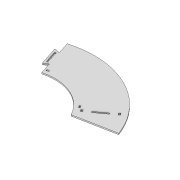
# Autodesk Inventor part: Level 1d - V2
Saved by Autodesk Inventor 2020 (Build 240168000, 168)
## iProperties
Created: 2020-07-30
Part Number: Level 1d - V2
Material: Generic
Document SubType Name: Modeling
Designer: Dan Wikman
Density: 1 g/cm^3
Appearance: Default
Author: Dan Wikman
Autodesk Inventor part; units mm, degrees
ref_plane "YZ Plane" through (0, 0, 0) normal (1, 0, 0) x (0, 1, 0)
ref_plane "XZ Plane" through (0, 0, 0) normal (0, 1, 0) x (-1, 0, 0)
ref_plane "XY Plane" through (0, 0, 0) normal (0, 0, 1) x (1, 0, 0)
sketch "Sketch1" plane through (0, 0, 0) normal (0, 1, 0) x (-1, 0, 0)
  line L0 (0, 0) -> (618.944217, 0)
  line L1 (0, 0) -> (191.264282, 588.650931)
  line L2 (0, 0) -> (-500.73639, 363.806283)
  line L3 (0, 0) -> (-500.73639, -363.806283)
  line L4 (0, 0) -> (191.264282, -588.650931)
  line L5 (396.643783, 3.75) -> (328.143784, 3.75)
  line L6 (328.143784, -3.75) -> (396.643784, -3.75)
  arc A0 (472.393783, 0) -> (145.977707, 449.273186) centre (0, 0) ccw
  arc A1 (77.993968, -240.040752) -> (252.393783, 0) centre (0, 0) ccw
  line L7 (289.893785, 3.75) -> (283.893784, 3.75)
  line L8 (283.893783, -3.75) -> (289.893781, -3.75)
  arc A2 (328.143784, 3.75) -> (326.393783, 2) centre (328.143783, 2) ccw
  arc A3 (326.393783, -1.999999) -> (328.143784, -3.75) centre (328.143783, -2) ccw
  line L9 (326.393783, 2) -> (326.393783, -1.999999)
  arc A4 (398.393783, 2) -> (396.643783, 3.75) centre (396.643783, 2) ccw
  arc A5 (396.643784, -3.75) -> (398.393783, -2.013555) centre (396.657285, -2.013555) ccw
  line L10 (398.393783, -2.013555) -> (398.393783, 2)
  line L11 (362.393784, -3.75) -> (362.393784, 32.980572)
  arc A6 (283.893784, 3.75) -> (282.143784, 2) centre (283.893784, 2) ccw
  arc A7 (282.143784, -2) -> (283.893783, -3.75) centre (283.893784, -2) ccw
  arc A8 (289.893781, -3.75) -> (291.643782, -2.000001) centre (289.893781, -2) ccw
  arc A9 (291.643784, 1.999999) -> (289.893785, 3.75) centre (289.893785, 2) ccw
  line L12 (291.643784, 1.999999) -> (291.643782, -2.000001)
  line L13 (282.143784, -2) -> (282.143784, 2)
  line L14 (434.893784, 3.75) -> (440.893785, 3.75)
  line L15 (440.893786, -3.75) -> (434.893788, -3.75)
  arc A10 (442.643785, 2) -> (440.893785, 3.75) centre (440.893785, 2) ccw
  arc A11 (440.893786, -3.75) -> (442.643785, -2) centre (440.893785, -2) ccw
  arc A12 (433.143787, -2.000001) -> (434.893788, -3.75) centre (434.893788, -2) ccw
  arc A13 (434.893784, 3.75) -> (433.143785, 1.999999) centre (434.893784, 2) ccw
  line L16 (433.143785, 1.999999) -> (433.143787, -2.000001)
  line L17 (442.643785, -2) -> (442.643785, 2)
  line L18 (131.946679, 412.562253) -> (135.750905, 411.326187)
  arc A14 (130.823108, 414.767381) -> (131.946679, 412.562253) centre (132.487457, 414.226602) ccw
  arc A15 (135.750905, 411.326187) -> (137.956033, 412.449757) centre (136.291684, 412.990537) ccw
  line L19 (139.810135, 418.156094) -> (137.956033, 412.449757)
  line L20 (130.823108, 414.767381) -> (132.67721, 420.473721)
  arc A16 (134.882339, 421.59729) -> (132.67721, 420.473721) centre (134.341559, 419.932941) ccw
  line L21 (138.686565, 420.361222) -> (134.882339, 421.59729)
  arc A17 (139.810135, 418.156094) -> (138.686565, 420.361222) centre (138.145785, 418.696873) ccw
  line L22 (125.025454, 378.272781) -> (121.208336, 379.513038)
  arc A18 (121.208336, 379.513038) -> (119.003208, 378.389469) centre (120.667557, 377.848689) ccw
  arc A19 (126.136132, 376.071842) -> (125.025454, 378.272781) centre (124.488846, 376.621273) ccw
  line L23 (119.003208, 378.389469) -> (97.835544, 313.242097)
  line L24 (98.959113, 311.036969) -> (102.763338, 309.800901)
  arc A20 (97.835544, 313.242097) -> (98.959113, 311.036969) centre (99.499893, 312.701317) ccw
  arc A21 (102.763338, 309.800901) -> (104.968468, 310.924471) centre (103.304119, 311.465249) ccw
  line L25 (104.968468, 310.924471) -> (126.136132, 376.071842)
  line L26 (88.220774, 277.987755) -> (92.024998, 276.751685)
  arc A22 (93.148567, 274.546556) -> (92.024998, 276.751685) centre (91.484218, 275.087336) ccw
  line L27 (91.294465, 268.840219) -> (93.148567, 274.546556)
  arc A23 (88.220774, 277.987755) -> (86.015644, 276.864187) centre (87.679993, 276.323407) ccw
  line L28 (86.015644, 276.864187) -> (84.161542, 271.157847)
  arc A24 (84.161542, 271.157847) -> (85.285111, 268.952718) centre (85.825891, 270.617067) ccw
  arc A25 (89.089337, 267.71665) -> (91.294465, 268.840219) centre (89.630117, 269.380999) ccw
  line L29 (89.089337, 267.71665) -> (85.285111, 268.952718)
  line L30 (-351.596253, 252.977496) -> (-349.245114, 256.213565)
  arc A26 (-354.040657, 252.590339) -> (-351.596253, 252.977496) centre (-353.012033, 254.006119) ccw
  arc A27 (-349.245114, 256.213565) -> (-349.63227, 258.657968) centre (-350.660895, 257.242188) ccw
  line L31 (-354.486371, 262.184679) -> (-349.63227, 258.657968)
  line L32 (-354.040657, 252.590339) -> (-358.89476, 256.117051)
  arc A28 (-359.281915, 258.561455) -> (-358.89476, 256.117051) centre (-357.866135, 257.532831) ccw
  line L33 (-356.930774, 261.797523) -> (-359.281915, 258.561455)
  arc A29 (-354.486371, 262.184679) -> (-356.930774, 261.797523) centre (-355.514994, 260.768899) ccw
  line L34 (-321.123804, 235.79899) -> (-323.482912, 232.551956)
  arc A30 (-323.482912, 232.551956) -> (-323.095756, 230.107553) centre (-322.067132, 231.523332) ccw
  arc A31 (-318.687368, 236.175181) -> (-321.123804, 235.79899) centre (-319.718947, 234.778302) ccw
  line L35 (-323.095756, 230.107553) -> (-267.678092, 189.844263)
  line L36 (-265.233688, 190.231418) -> (-262.882548, 193.467485)
  arc A32 (-267.678092, 189.844263) -> (-265.233688, 190.231418) centre (-266.649468, 191.260043) ccw
  arc A33 (-262.882548, 193.467485) -> (-263.269704, 195.911891) centre (-264.298327, 194.496111) ccw
  line L37 (-263.269704, 195.911891) -> (-318.687368, 236.175181)
  line L38 (-237.120347, 169.805882) -> (-234.769205, 173.041948)
  arc A34 (-232.324801, 173.429103) -> (-234.769205, 173.041948) centre (-233.353425, 172.013323) ccw
  line L39 (-227.4707, 169.902393) -> (-232.324801, 173.429103)
  arc A35 (-237.120347, 169.805882) -> (-236.733193, 167.361478) centre (-235.704569, 168.777257) ccw
  line L40 (-236.733193, 167.361478) -> (-231.87909, 163.834766)
  arc A36 (-231.87909, 163.834766) -> (-229.434686, 164.221921) centre (-230.850466, 165.250545) ccw
  arc A37 (-227.083545, 167.457989) -> (-227.4707, 169.902393) centre (-228.499325, 168.486613) ccw
  line L41 (-227.083545, 167.457989) -> (-229.434686, 164.221921)
  line L42 (-349.245113, -256.213562) -> (-351.596256, -252.977496)
  arc A38 (-349.632267, -258.657966) -> (-349.245113, -256.213562) centre (-350.660892, -257.242187) ccw
  arc A39 (-351.596256, -252.977496) -> (-354.04066, -252.590341) centre (-353.012035, -254.006121) ccw
  line L43 (-358.89476, -256.117051) -> (-354.04066, -252.590341)
  line L44 (-349.632267, -258.657966) -> (-354.48637, -262.184678)
  arc A40 (-356.930774, -261.797523) -> (-354.48637, -262.184678) centre (-355.514994, -260.768899) ccw
  line L45 (-359.281915, -258.561455) -> (-356.930774, -261.797523)
  arc A41 (-358.89476, -256.117051) -> (-359.281915, -258.561455) centre (-357.866135, -257.532831) ccw
  line L46 (-323.490879, -232.540991) -> (-321.131771, -235.788024)
  arc A42 (-321.131771, -235.788024) -> (-318.687367, -236.17518) centre (-319.715991, -234.7594) ccw
  arc A43 (-323.095757, -230.107553) -> (-323.490879, -232.540991) centre (-322.086023, -231.520303) ccw
  line L47 (-318.687367, -236.17518) -> (-263.269703, -195.91189)
  line L48 (-262.882547, -193.467486) -> (-265.233687, -190.231419)
  arc A44 (-263.269703, -195.91189) -> (-262.882547, -193.467486) centre (-264.298327, -194.496111) ccw
  arc A45 (-265.233687, -190.231419) -> (-267.678093, -189.844263) centre (-266.649468, -191.260043) ccw
  line L49 (-267.678093, -189.844263) -> (-323.095757, -230.107553)
  line L50 (-234.769208, -173.041948) -> (-237.120347, -169.805879)
  arc A46 (-236.73319, -167.361476) -> (-237.120347, -169.805879) centre (-235.704566, -168.777256) ccw
  line L51 (-231.87909, -163.834765) -> (-236.73319, -167.361476)
  arc A47 (-234.769208, -173.041948) -> (-232.324804, -173.429105) centre (-233.353428, -172.013326) ccw
  line L52 (-232.324804, -173.429105) -> (-227.470701, -169.902393)
  arc A48 (-227.470701, -169.902393) -> (-227.083545, -167.457989) centre (-228.499325, -168.486613) ccw
  arc A49 (-229.434686, -164.221921) -> (-231.87909, -163.834765) centre (-230.850466, -165.250545) ccw
  line L53 (-229.434686, -164.221921) -> (-227.083545, -167.457989)
  line L54 (135.750902, -411.326185) -> (131.946678, -412.562255)
  arc A50 (137.956032, -412.449754) -> (135.750902, -411.326185) centre (136.291683, -412.990533) ccw
  arc A51 (131.946678, -412.562255) -> (130.823109, -414.767384) centre (132.487459, -414.226604) ccw
  line L55 (132.677211, -420.473722) -> (130.823109, -414.767384)
  line L56 (137.956032, -412.449754) -> (139.810134, -418.156094)
  arc A52 (138.686565, -420.361222) -> (139.810134, -418.156094) centre (138.145785, -418.696873) ccw
  line L57 (134.882339, -421.59729) -> (138.686565, -420.361222)
  arc A53 (132.677211, -420.473722) -> (134.882339, -421.59729) centre (134.341559, -419.932941) ccw
  line L58 (121.195445, -379.517226) -> (125.012563, -378.27697)
  arc A54 (125.012563, -378.27697) -> (126.136132, -376.071841) centre (124.471783, -376.612621) ccw
  arc A55 (119.003208, -378.38947) -> (121.195445, -379.517226) centre (120.658838, -377.865719) ccw
  line L59 (126.136132, -376.071841) -> (104.968468, -310.92447)
  line L60 (102.763339, -309.800901) -> (98.959114, -311.036968)
  arc A56 (104.968468, -310.92447) -> (102.763339, -309.800901) centre (103.304119, -311.465249) ccw
  arc A57 (98.959114, -311.036968) -> (97.835544, -313.242098) centre (99.499893, -312.701317) ccw
  line L61 (97.835544, -313.242098) -> (119.003208, -378.38947)
  line L62 (92.024997, -276.751688) -> (88.220771, -277.987753)
  arc A58 (86.015643, -276.864184) -> (88.220771, -277.987753) centre (87.679992, -276.323404) ccw
  line L63 (84.161542, -271.157846) -> (86.015643, -276.864184)
  arc A59 (92.024997, -276.751688) -> (93.148568, -274.546559) centre (91.484219, -275.087339) ccw
  line L64 (93.148568, -274.546559) -> (91.294466, -268.840219)
  arc A60 (91.294466, -268.840219) -> (89.089337, -267.71665) centre (89.630117, -269.380999) ccw
  arc A61 (85.285111, -268.952718) -> (84.161542, -271.157846) centre (85.825891, -270.617067) ccw
  line L65 (85.285111, -268.952718) -> (89.089337, -267.71665)
  line L66 (-442.530326, 165.296089) -> (-220.837003, 122.203273)
  line L67 (-442.530326, -165.296089) -> (-220.837003, -122.203273)
  arc A62 (252.393783, 0) -> (-220.837003, 122.203273) centre (0, 0) ccw
  arc A63 (-220.837003, -122.203273) -> (77.993968, -240.040752) centre (0, 0) ccw
  arc A64 (145.977707, 449.273186) -> (-442.530326, 165.296089) centre (0, 0) ccw
  arc A65 (-442.530326, -165.296089) -> (472.393783, 0) centre (0, 0) ccw
  line L68 (115.678154, 400.516685) -> (82.986198, 299.90119)
  line L69 (84.650547, 297.61041) -> (108.748421, 297.61041)
  line L70 (110.41277, 295.31963) -> (90.955171, 235.435297)
  line L71 (138.866228, 382.890368) -> (158.992883, 444.833845)
  line L72 (118.634381, 401.156393) -> (135.910001, 382.25066)
  line L73 (123.116895, 378.892909) -> (127.272191, 391.703526) construction
  line L74 (100.861225, 310.418935) -> (96.699484, 297.61041) construction
  arc A66 (135.910001, 382.25066) -> (138.866228, 382.890368) centre (137.201879, 383.431148) ccw
  arc A67 (118.634381, 401.156393) -> (115.678154, 400.516685) centre (117.342503, 399.975905) ccw
  arc A68 (82.986198, 299.90119) -> (84.650547, 297.61041) centre (84.650547, 299.36041) ccw
  arc A69 (110.41277, 295.31963) -> (108.748421, 297.61041) centre (108.748421, 295.86041) ccw
  line L75 (407.062404, -13.75) -> (472.19363, -13.75)
  arc A70 (405.540481, -11.136142) -> (407.062404, -13.75) centre (407.062404, -12) ccw
  line L76 (418.182442, 11.136142) -> (405.540481, -11.136142)
  arc A71 (418.182442, 11.136142) -> (416.660519, 13.75) centre (416.660519, 12) ccw
  line L77 (416.660519, 13.75) -> (310.867126, 13.75)
  line L78 (309.202778, 11.45922) -> (316.64943, -11.45922)
  arc A72 (310.867126, 13.75) -> (309.202778, 11.45922) centre (310.867126, 12) ccw
  arc A73 (314.985081, -13.75) -> (316.64943, -11.45922) centre (314.985081, -12) ccw
  line L79 (314.985081, -13.75) -> (252.018966, -13.75)
  line L80 (112.712173, -391.388335) -> (132.838829, -453.331812)
  arc A74 (114.7278, -389.133174) -> (112.712173, -391.388335) centre (114.376522, -390.847556) ccw
  line L81 (139.816582, -394.273879) -> (114.7278, -389.133174)
  arc A75 (139.816582, -394.273879) -> (141.832208, -392.018718) centre (140.167859, -392.559497) ccw
  line L82 (141.832208, -392.018718) -> (109.140252, -291.403223)
  line L83 (106.447279, -290.528223) -> (86.951689, -304.692598)
  arc A76 (109.140252, -291.403223) -> (106.447279, -290.528223) centre (107.475903, -291.944002) ccw
  arc A77 (84.258716, -303.817598) -> (86.951689, -304.692598) centre (85.923065, -303.276818) ccw
  line L84 (84.258716, -303.817598) -> (64.801116, -243.933264)
  line L85 (277, 35.5) -> (273, 35.5)
  line L86 (271.25, 33.75) -> (271.25, 23.75)
  line L87 (273, 22) -> (277, 22)
  line L88 (278.75, 23.75) -> (278.75, 33.75)
  arc A78 (278.75, 33.75) -> (277, 35.5) centre (277, 33.75) ccw
  arc A79 (273, 35.5) -> (271.25, 33.75) centre (273, 33.75) ccw
  arc A80 (271.25, 23.75) -> (273, 22) centre (273, 23.75) ccw
  arc A81 (277, 22) -> (278.75, 23.75) centre (277, 23.75) ccw
  line L89 (277, -35.5) -> (273, -35.5)
  line L90 (271.25, -33.75) -> (271.25, -23.75)
  line L91 (273, -22) -> (277, -22)
  line L92 (278.75, -23.75) -> (278.75, -33.75)
  arc A82 (277, -35.5) -> (278.75, -33.75) centre (277, -33.75) ccw
  arc A83 (271.25, -33.75) -> (273, -35.5) centre (273, -33.75) ccw
  arc A84 (273, -22) -> (271.25, -23.75) centre (273, -23.75) ccw
  arc A85 (278.75, -23.75) -> (277, -22) centre (277, -23.75) ccw
  arc A86 (64.674464, 270.241029) -> (63.550895, 272.446158) centre (63.010115, 270.781809) ccw
  line L93 (63.550895, 272.446158) -> (54.04033, 275.536327)
  line L94 (63.438396, 266.436803) -> (64.674464, 270.241029)
  arc A87 (61.233267, 265.313234) -> (63.438396, 266.436803) centre (61.774047, 266.977583) ccw
  line L95 (51.835201, 274.412758) -> (50.599133, 270.608532)
  line L96 (51.722702, 268.403404) -> (61.233267, 265.313234)
  arc A88 (50.599133, 270.608532) -> (51.722702, 268.403404) centre (52.263482, 270.067753) ccw
  arc A89 (54.04033, 275.536327) -> (51.835201, 274.412758) centre (53.49955, 273.871979) ccw
  arc A90 (108.726079, 257.76785) -> (106.520951, 256.644281) centre (108.1853, 256.103501) ccw
  line L97 (105.284883, 252.840055) -> (106.520951, 256.644281)
  arc A91 (105.284883, 252.840055) -> (106.408452, 250.634926) centre (106.949232, 252.299275) ccw
  line L98 (108.726079, 257.76785) -> (118.236645, 254.67768)
  arc A92 (119.360214, 252.472552) -> (118.236645, 254.67768) centre (117.695865, 253.013331) ccw
  line L99 (115.919017, 247.544756) -> (106.408452, 250.634926)
  line L100 (119.360214, 252.472552) -> (118.124146, 248.668326)
  arc A93 (115.919017, 247.544756) -> (118.124146, 248.668326) centre (116.459797, 249.209105) ccw
  arc A94 (-211.553587, 183.059293) -> (-211.166432, 180.614889) centre (-210.137808, 182.030669) ccw
  line L101 (-207.930364, 178.263748) -> (-211.166432, 180.614889)
  arc A95 (-207.930364, 178.263748) -> (-205.48596, 178.650903) centre (-206.90174, 179.679527) ccw
  line L102 (-211.553587, 183.059293) -> (-205.675735, 191.149463)
  arc A96 (-203.231331, 191.536618) -> (-205.675735, 191.149463) centre (-204.259955, 190.120838) ccw
  line L103 (-199.608107, 186.741073) -> (-205.48596, 178.650903)
  line L104 (-203.231331, 191.536618) -> (-199.995263, 189.185477)
  arc A97 (-199.608107, 186.741073) -> (-199.995263, 189.185477) centre (-201.023887, 187.769697) ccw
  arc A98 (-211.166432, -180.614889) -> (-211.553587, -183.059293) centre (-210.137808, -182.030669) ccw
  line L105 (-211.553587, -183.059293) -> (-205.675735, -191.149463)
  line L106 (-207.930364, -178.263748) -> (-211.166432, -180.614889)
  arc A99 (-205.48596, -178.650903) -> (-207.930364, -178.263748) centre (-206.90174, -179.679527) ccw
  line L107 (-203.231331, -191.536618) -> (-199.995263, -189.185477)
  line L108 (-199.608107, -186.741073) -> (-205.48596, -178.650903)
  arc A100 (-199.995263, -189.185477) -> (-199.608107, -186.741073) centre (-201.023887, -187.769697) ccw
  arc A101 (-205.675735, -191.149463) -> (-203.231331, -191.536618) centre (-204.259955, -190.120838) ccw
  arc A102 (106.520951, -256.644281) -> (108.726079, -257.76785) centre (108.1853, -256.103501) ccw
  line L109 (108.726079, -257.76785) -> (118.236645, -254.67768)
  line L110 (105.284883, -252.840055) -> (106.520951, -256.644281)
  arc A103 (106.408452, -250.634926) -> (105.284883, -252.840055) centre (106.949232, -252.299275) ccw
  line L111 (119.360214, -252.472552) -> (118.124146, -248.668326)
  line L112 (115.919017, -247.544756) -> (106.408452, -250.634926)
  arc A104 (118.124146, -248.668326) -> (115.919017, -247.544756) centre (116.459797, -249.209105) ccw
  arc A105 (118.236645, -254.67768) -> (119.360214, -252.472552) centre (117.695865, -253.013331) ccw
  arc A106 (63.550895, -272.446158) -> (64.674464, -270.241029) centre (63.010115, -270.781809) ccw
  line L113 (63.438396, -266.436803) -> (64.674464, -270.241029)
  arc A107 (63.438396, -266.436803) -> (61.233267, -265.313234) centre (61.774047, -266.977583) ccw
  line L114 (63.550895, -272.446158) -> (54.04033, -275.536327)
  arc A108 (51.835201, -274.412758) -> (54.04033, -275.536327) centre (53.49955, -273.871979) ccw
  line L115 (51.722702, -268.403404) -> (61.233267, -265.313234)
  line L116 (51.835201, -274.412758) -> (50.599133, -270.608532)
  arc A109 (51.722702, -268.403404) -> (50.599133, -270.608532) centre (52.263482, -270.067753) ccw
  line L117 (-351.596253, 252.977496) -> (-355.245358, 247.912443)
  line L118 (-359.281915, 258.561455) -> (-362.91513, 253.454684)
  line L119 (-357.693866, 247.519615) -> (-362.517811, 251.024417)
  arc A110 (-362.91513, 253.454684) -> (-362.517811, 251.024417) centre (-361.489187, 252.440196) ccw
  arc A111 (-357.693866, 247.519615) -> (-355.245358, 247.912443) centre (-356.665241, 248.935395) ccw
  line L120 (-229.434685, 164.221921) -> (-233.08379, 159.156869)
  line L121 (-237.120347, 169.805881) -> (-240.753562, 164.69911)
  line L122 (-235.532298, 158.764041) -> (-240.356243, 162.268842)
  arc A112 (-240.753562, 164.69911) -> (-240.356243, 162.268842) centre (-239.327619, 163.684622) ccw
  arc A113 (-235.532298, 158.764041) -> (-233.08379, 159.156869) centre (-234.503673, 160.17982) ccw
  line L123 (-223.777058, -174.94374) -> (-228.601004, -178.448542)
  line L124 (-234.769206, -173.041949) -> (-231.035104, -178.07542)
  arc A114 (-231.035104, -178.07542) -> (-228.601004, -178.448542) centre (-229.629628, -177.032762) ccw
  arc A115 (-223.777058, -174.94374) -> (-223.394029, -172.49368) centre (-224.805682, -173.52796) ccw
  line L125 (-227.083545, -167.457988) -> (-223.394029, -172.49368)
  line L126 (97.23047, -266.885218) -> (99.073053, -272.556106)
  line L127 (92.024998, -276.751686) -> (97.966015, -274.755772)
  arc A116 (97.966015, -274.755772) -> (99.073053, -272.556106) centre (97.408704, -273.096886) ccw
  arc A117 (97.23047, -266.885218) -> (95.018687, -265.763826) centre (95.566121, -267.425998) ccw
  line L128 (89.089336, -267.716649) -> (95.018687, -265.763826)
  line L129 (283.868793, 9.999604) -> (289.831518, 9.999604)
  line L130 (291.643783, 2) -> (291.581431, 8.267014)
  arc A118 (291.581431, 8.267014) -> (289.831518, 9.999604) centre (289.831518, 8.249604) ccw
  arc A119 (283.868793, 9.999604) -> (282.118807, 8.242603) centre (283.868793, 8.249604) ccw
  line L131 (282.143783, 1.999999) -> (282.118807, 8.242603)
  line L132 (78.210093, 273.065313) -> (80.052676, 278.736201)
  line L133 (88.220772, 277.987754) -> (82.24122, 279.865068)
  arc A120 (82.24122, 279.865068) -> (80.052676, 278.736201) centre (81.717025, 278.195422) ccw
  arc A121 (78.210093, 273.065313) -> (79.340325, 270.858034) centre (79.874441, 272.524533) ccw
  line L134 (85.285111, 268.952717) -> (79.340325, 270.858034)
  line L135 (-356.930774, -261.797523) -> (-353.196672, -266.830994)
  arc A122 (-353.196672, -266.830994) -> (-350.762571, -267.204116) centre (-351.791195, -265.788336) ccw
  line L136 (-345.938626, -263.699314) -> (-350.762571, -267.204116)
  arc A123 (-345.938626, -263.699314) -> (-345.555597, -261.249254) centre (-346.96725, -262.283534) ccw
  line L137 (-349.245112, -256.213562) -> (-345.555597, -261.249254)
  line L138 (138.686565, -420.361222) -> (144.627582, -418.365308)
  arc A124 (144.627582, -418.365308) -> (145.73462, -416.165642) centre (144.070271, -416.706422) ccw
  line L139 (143.892037, -410.494753) -> (145.73462, -416.165642)
  arc A125 (143.892037, -410.494753) -> (141.680254, -409.373361) centre (142.227688, -411.035533) ccw
  line L140 (135.750903, -411.326185) -> (141.680254, -409.373361)
  line L141 (442.643785, 2) -> (442.581433, 8.267014)
  arc A126 (442.581433, 8.267014) -> (440.83152, 9.999604) centre (440.83152, 8.249604) ccw
  line L142 (434.868795, 9.999604) -> (440.83152, 9.999604)
  arc A127 (434.868795, 9.999604) -> (433.118809, 8.242603) centre (434.868795, 8.249604) ccw
  line L143 (433.143784, 1.999999) -> (433.118809, 8.242603)
  line L144 (134.882339, 421.59729) -> (128.902786, 423.474604)
  arc A128 (128.902786, 423.474604) -> (126.714243, 422.345737) centre (128.378591, 421.804957) ccw
  line L145 (124.871659, 416.674849) -> (126.714243, 422.345737)
  arc A129 (124.871659, 416.674849) -> (126.001891, 414.46757) centre (126.536008, 416.134069) ccw
  line L146 (131.946678, 412.562252) -> (126.001891, 414.46757)
  point P0 (115.5523, 343.498156)
  point P1 (-290.978536, 216.043536)
  point P2 (-295.386925, -209.975908)
  point P3 (108.419376, -345.815784)
  point P4 (137.937454, 380.031898)
  point P5 (97.940631, 311.906834)
  point P6 (104.098602, 309.905988)
  point P7 (119.873073, 379.40795)
  point P8 (404.05683, -13.75)
  point P9 (411.861461, 0)
  point P10 (312.926104, 0)
  point P11 (111.7834, -388.529865)
  point P12 (127.272191, -391.703526)
  point P13 (96.699484, -297.61041)
  point P14 (-363.919575, 252.042858)
  point P15 (-359.302101, 258.533082)
  point P16 (-352.164335, -268.222557)
  point P17 (146.270046, -417.813514)
  point P18 (442.564195, 9.999604)
  point P19 (127.249669, 423.993609)
  point P20 (85.285111, 268.952717)
  point P21 (88.187448, 277.998217)
  point P22 (-229.434685, 164.22192)
  point P23 (-237.140595, 169.77742)
  point P24 (131.946678, 412.562252)
  point P25 (134.849097, 421.607727)
  point P26 (282.143782, 2)
  point P27 (291.643436, 2.034926)
  point P28 (433.143784, 1.999999)
  point P29 (442.643438, 2.03484)
  point P30 (89.089337, -267.716648)
  point P31 (92.058108, -276.740563)
  point P32 (135.750902, -411.326185)
  point P33 (138.719593, -420.350126)
  point P34 (-349.245113, -256.213562)
  point P35 (-356.910015, -261.825505)
  point P36 (-227.083546, -167.457989)
  point P37 (-234.748396, -173.07)
  dimension "d4" = 360
  dimension "d6" = 7.5
  dimension "d7" = 7.5
  dimension "d9" = 68.5
  dimension "d10" = 7.5
  dimension "d11" = 7.5
  dimension "d12" = 3.5
  dimension "d13" = 3.5
  dimension "d19" = 360
  dimension "d21" = 25
  dimension "d25" = 10
  dimension "d26" = 10
  dimension "d27" = 1.75
  dimension "d30" = 144
  dimension "d32" = 271.25
  dimension "d33" = 7.5
  dimension "d34" = 13.5
  dimension "d36" = 1.75
  dimension "d40" = 20
  dimension "d46" = 0
  dimension "d47" = 8
  dimension "d48" = 1.75
  dimension "d67" = 1.75
  constraints: 294 end point, 265 point on circle, 130 centre point, 30 tangent, 26 point on line, 26 symmetric about line, 8 equal radius, 6 parallel, 5 horizontal, 5 midpoint, 2 coincident, 2 vertical, 1 equal length, 1 perpendicular, 390 other
  measures "d6" distance between parallel lines of L5 L6
  measures "d7" diameter of L6 L0
  measures "d9" distance of L6.start L6.end
  measures "d10" distance between parallel lines of L7 L8
  measures "d11" diameter of L7 L0
  measures "d12" diameter of A2
  measures "d13" diameter of A3
  measures "d21" angle of L35 L66
  measures "d25" distance between parallel lines of L23 L68
  measures "d26" distance between parallel lines of L25 L70
  measures "d27" radius of A66
  measures "d32" distance from line of point (0, 0) L86
  measures "d33" distance between parallel lines of L86 L88
  measures "d34" distance between parallel lines of L85 L87
  measures "d36" radius of A78
  measures "d40" distance from line of L5 A81.centre
  measures "d46" angle of L32 L119
  measures "d47" distance of L33.end point (-363.92, 252.043)
  measures "d48" radius of A110
  measures "d67" radius of A112
sketch "Sketch1 outline for Extrusion1" plane through (0, 0, 0) normal (0, 1, 0) x (-1, 0, 0)
  line L0 (106.447279, -290.528223) -> (86.951689, -304.692598)
  arc A0 (109.140252, -291.403223) -> (106.447279, -290.528223) centre (107.475903, -291.944002) ccw
  arc A1 (86.951689, -304.692598) -> (84.258716, -303.817598) centre (85.923065, -303.276818) cw
  line L1 (141.832208, -392.018718) -> (109.140252, -291.403223)
  line L2 (84.258716, -303.817598) -> (64.801116, -243.933264)
  arc A2 (139.816582, -394.273879) -> (141.832208, -392.018718) centre (140.167859, -392.559497) ccw
  arc A3 (64.801116, -243.933264) -> (-220.837003, -122.203273) centre (0, 0) cw
  line L3 (114.7278, -389.133174) -> (139.816582, -394.273879)
  line L4 (-220.837003, -122.203273) -> (-442.530326, -165.296089)
  arc A4 (112.712173, -391.388335) -> (114.7278, -389.133174) centre (114.376522, -390.847556) cw
  arc A5 (-442.530326, -165.296089) -> (132.838829, -453.331812) centre (0, 0) ccw
  line L5 (132.838829, -453.331812) -> (112.712173, -391.388335)
  line L6 (98.959114, -311.036968) -> (102.763339, -309.800901)
  arc A6 (97.835544, -313.242098) -> (98.959114, -311.036968) centre (99.499893, -312.701317) cw
  line L7 (119.003208, -378.38947) -> (97.835544, -313.242098)
  arc A7 (121.195445, -379.517226) -> (119.003208, -378.38947) centre (120.658838, -377.865719) cw
  line L8 (125.012563, -378.27697) -> (121.195445, -379.517226)
  arc A8 (126.136132, -376.071841) -> (125.012563, -378.27697) centre (124.471783, -376.612621) cw
  line L9 (104.968468, -310.92447) -> (126.136132, -376.071841)
  arc A9 (102.763339, -309.800901) -> (104.968468, -310.92447) centre (103.304119, -311.465249) cw
  line L10 (-351.596256, -252.977496) -> (-349.245113, -256.213562)
  arc A10 (-354.04066, -252.590341) -> (-351.596256, -252.977496) centre (-353.012035, -254.006121) cw
  line L11 (-358.89476, -256.117051) -> (-354.04066, -252.590341)
  arc A11 (-359.281915, -258.561455) -> (-358.89476, -256.117051) centre (-357.866135, -257.532831) cw
  line L12 (-356.930774, -261.797523) -> (-359.281915, -258.561455)
  arc A12 (-356.910015, -261.825505) -> (-356.930774, -261.797523) centre (-355.514994, -260.768899) cw
  line L13 (-353.196672, -266.830994) -> (-356.910015, -261.825505)
  arc A13 (-350.762571, -267.204116) -> (-353.196672, -266.830994) centre (-351.791195, -265.788336) cw
  line L14 (-345.938626, -263.699314) -> (-350.762571, -267.204116)
  arc A14 (-345.555597, -261.249254) -> (-345.938626, -263.699314) centre (-346.96725, -262.283534) cw
  line L15 (-349.245113, -256.213562) -> (-345.555597, -261.249254)
  line L16 (-321.131771, -235.788024) -> (-323.490879, -232.540991)
  arc A15 (-318.687367, -236.17518) -> (-321.131771, -235.788024) centre (-319.715991, -234.7594) cw
  line L17 (-263.269703, -195.91189) -> (-318.687367, -236.17518)
  arc A16 (-262.882547, -193.467486) -> (-263.269703, -195.91189) centre (-264.298327, -194.496111) cw
  line L18 (-265.233687, -190.231419) -> (-262.882547, -193.467486)
  arc A17 (-267.678093, -189.844263) -> (-265.233687, -190.231419) centre (-266.649468, -191.260043) cw
  line L19 (-323.095757, -230.107553) -> (-267.678093, -189.844263)
  arc A18 (-323.490879, -232.540991) -> (-323.095757, -230.107553) centre (-322.086023, -231.520303) cw
  line L20 (-205.48596, -178.650903) -> (-199.608107, -186.741073)
  arc A19 (-207.930364, -178.263748) -> (-205.48596, -178.650903) centre (-206.90174, -179.679527) cw
  line L21 (-211.166432, -180.614889) -> (-207.930364, -178.263748)
  arc A20 (-211.553587, -183.059293) -> (-211.166432, -180.614889) centre (-210.137808, -182.030669) cw
  line L22 (-205.675735, -191.149463) -> (-211.553587, -183.059293)
  arc A21 (-203.231331, -191.536618) -> (-205.675735, -191.149463) centre (-204.259955, -190.120838) cw
  line L23 (-199.995263, -189.185477) -> (-203.231331, -191.536618)
  arc A22 (-199.608107, -186.741073) -> (-199.995263, -189.185477) centre (-201.023887, -187.769697) cw
  line L24 (-229.434686, -164.221921) -> (-227.083546, -167.457989)
  arc A23 (-231.87909, -163.834765) -> (-229.434686, -164.221921) centre (-230.850466, -165.250545) cw
  line L25 (-236.73319, -167.361476) -> (-231.87909, -163.834765)
  arc A24 (-237.120347, -169.805879) -> (-236.73319, -167.361476) centre (-235.704566, -168.777256) cw
  line L26 (-234.769208, -173.041948) -> (-237.120347, -169.805879)
  arc A25 (-234.748396, -173.07) -> (-234.769208, -173.041948) centre (-233.353428, -172.013326) cw
  line L27 (-231.035104, -178.07542) -> (-234.748396, -173.07)
  arc A26 (-228.601004, -178.448542) -> (-231.035104, -178.07542) centre (-229.629628, -177.032762) cw
  line L28 (-223.777058, -174.94374) -> (-228.601004, -178.448542)
  arc A27 (-223.394029, -172.49368) -> (-223.777058, -174.94374) centre (-224.805682, -173.52796) cw
  line L29 (-227.083546, -167.457989) -> (-223.394029, -172.49368)
  line L30 (51.835201, -274.412758) -> (50.599133, -270.608532)
  arc A28 (54.04033, -275.536327) -> (51.835201, -274.412758) centre (53.49955, -273.871979) cw
  line L31 (63.550895, -272.446158) -> (54.04033, -275.536327)
  arc A29 (64.674464, -270.241029) -> (63.550895, -272.446158) centre (63.010115, -270.781809) cw
  line L32 (63.438396, -266.436803) -> (64.674464, -270.241029)
  arc A30 (61.233267, -265.313234) -> (63.438396, -266.436803) centre (61.774047, -266.977583) cw
  line L33 (51.722702, -268.403404) -> (61.233267, -265.313234)
  arc A31 (50.599133, -270.608532) -> (51.722702, -268.403404) centre (52.263482, -270.067753) cw
extrude "Extrusion1" add sketch "Sketch1 outline for Extrusion1" along normal blind 7
body "Solid1"
